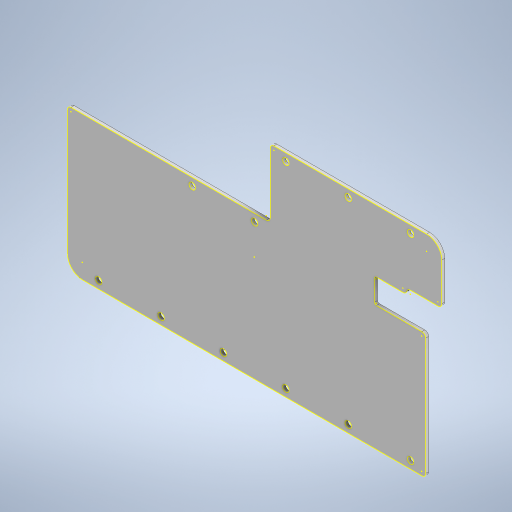
# Autodesk Inventor part: Class-D RevA Board Outline
Saved by Autodesk Inventor 2024 (Build 280153000, 153)
## iProperties
Created: 2023-08-05
Part Number: Class-D RevA Board Outline
Material: Generic
Document SubType Name: Modeling
Designer: Ishaan
Density: 1 g/cm^3
Appearance: Default
Author: Ishaan
Autodesk Inventor part; units mm, degrees
ref_plane "YZ Plane" through (0, 0, 0) normal (1, 0, 0) x (0, 1, 0)
ref_plane "XZ Plane" through (0, 0, 0) normal (0, 1, 0) x (-1, 0, 0)
ref_plane "XY Plane" through (0, 0, 0) normal (0, 0, 1) x (1, 0, 0)
sketch "Sketch1" plane through (0, 0, 0) normal (0, 0, 1) x (1, 0, 0)
  line L0 (-99, -56) -> (99, -56)
  line L1 (99, -56) -> (99, 56)
  line L2 (99, 56) -> (-99, 56)
  line L3 (-99, 56) -> (-99, -56)
  line L4 (-99, -56) -> (99, 56) construction
  line L5 (99, -56) -> (-99, 56) construction
  line L6 (-99, -56) -> (8.25, -56)
  line L7 (8.25, -56) -> (8.25, 20)
  line L8 (8.25, 20) -> (-99, 20)
  line L9 (-99, 20) -> (-99, -56)
  line L10 (8.25, 20) -> (8.25, 56)
  point P0 (0, 0)
  dimension "d0" = 112
  dimension "d1" = 198
  dimension "d3" = 76
  dimension "d50" = 8.25
  constraints: 22 end point, 4 parallel, 3 perpendicular, 2 horizontal, 2 midpoint, 1 point on line
  measures "d0" distance of L0.end L1.end
  measures "d1" distance of L1.end L2.end
  measures "d3" distance of L6.end L7.end
  measures "d50" distance from line of L10 point (0, 0)
extrude "Extrusion1" add sketch "Sketch1" along normal blind 1.6 contours L3 L8 L7 L0 | L7 L10 L2 L1 L0
sketch "Sketch2" plane through (0, 0, 1.6) normal (0, 0, 1) x (1, 0, 0)
  line L0 (-99, -56) -> (99, -56) projected
  line L1 (-99, 20) -> (-99, -56) projected
  line L2 (99, 56) -> (8.25, 56) projected
  line L3 (99, -56) -> (99, 56) projected
  line L4 (8.25, 20) -> (-99, 20) projected
  line L5 (-16.5, -52) -> (16.5, -52) construction
  line L6 (-49.5, -52) -> (-16.5, -52) construction
  point P0 (0, 0)
  point P1 (-82.5, -52)
  point P2 (49.5, -52)
  point P3 (-82.5, 52)
  point P4 (-49.5, 52)
  point P5 (-16.5, 52)
  point P6 (16.5, 52)
  point P7 (49.5, 52)
  point P8 (82.5, -52)
  point P9 (82.5, 52)
  point P10 (-33, 16)
  point P11 (0, 16)
  point P12 (0, -52)
  point P13 (-33, -52)
  point P14 (-99, 56)
  dimension "d6" = 4
  dimension "d9" = 33
  dimension "d12" = 104
  dimension "d15" = 4
  dimension "d17" = 16.5
  dimension "d18" = 16.5
  dimension "d26" = 4
  constraints: 4 end point, 3 horizontal, 2 midpoint, 2 vertical alignment, 1 coincident, 1 horizontal alignment, 1 vertical, 11 other
  measures "d6" distance from line of point (-82.5, -52) L0
  measures "d9" distance of point (-82.5, -52) L6.start
  measures "d12" distance of point (-82.5, -52) point (-82.5, 52)
  measures "d15" distance from line of L2 point (-82.5, 52)
  measures "d17" distance from line of point (-82.5, -52) L1
  measures "d18" distance from line of point (82.5, -52) L3
  measures "d26" distance from line of L4 point (-33, 16)
hole "Hole1" at (-82.5, -52, 1.6) at (-49.5, -52, 1.6) at (-16.5, -52, 1.6) at (16.5, -52, 1.6) at (49.5, -52, 1.6) at (-82.5, 52, 1.6) at (-49.5, 52, 1.6) at (-16.5, 52, 1.6) at (16.5, 52, 1.6) at (49.5, 52, 1.6) at (82.5, -52, 1.6) at (82.5, 52, 1.6) at (-33, 16, 1.6) at (0, 16, 1.6) direction (0, 0, -1) diameter 3.4 end through all
sketch "Sketch3" plane through (0, 0, 1.6) normal (0, 0, 1) x (1, 0, 0)
  circle A0 centre (0, 16) radius 1.7 projected
  circle A1 centre (-33, 16) radius 1.7 projected
  circle A2 centre (82.5, 52) radius 1.7 projected
  circle A3 centre (82.5, -52) radius 1.7 projected
  circle A4 centre (49.5, 52) radius 1.7 projected
  circle A5 centre (16.5, 52) radius 1.7 projected
  circle A6 centre (49.5, -52) radius 1.7 projected
  circle A7 centre (16.5, -52) radius 1.7 projected
  circle A8 centre (-16.5, -52) radius 1.7 projected
  circle A9 centre (-49.5, -52) radius 1.7 projected
  circle A10 centre (-82.5, -52) radius 1.7 projected
  line L0 (99, 56) -> (8.25, 56) projected
  line L1 (-99, 20) -> (-99, -56) projected
  line L2 (-99, -56) -> (99, -56) projected
  line L3 (99, -56) -> (99, 56) projected
  line L4 (99, 26) -> (0, 26) construction
  line L5 (99, 10) -> (-99, 10) construction
  line L6 (90.5, -56) -> (90.5, 10)
  line L7 (99, 26) -> (80.5, 26)
  line L8 (80.5, 26) -> (80.5, 10)
  line L9 (90.5, 10) -> (80.5, 10)
  line L10 (63.5, 10) -> (80.5, 10)
  line L11 (80.5, 10) -> (80.5, 23)
  line L12 (80.5, 23) -> (63.5, 23)
  line L13 (63.5, 23) -> (63.5, 10)
  line L14 (63.5, 10) -> (80.5, 23) construction
  line L15 (80.5, 10) -> (63.5, 23) construction
  line L16 (8.25, 56) -> (8.25, 20) projected
  line L17 (8.25, 20) -> (-99, 20) projected
  point P0 (0, 0)
  point P1 (82.5, 30)
  point P2 (72, 16.5)
  dimension "d27" = 30
  dimension "d29" = 4
  dimension "d30" = 8
  dimension "d31" = 4
  dimension "d32" = 4
  dimension "d33" = 2
  dimension "d36" = 72.5
  dimension "d37" = 17
  dimension "d38" = 13
  constraints: 24 end point, 8 point on line, 3 perpendicular, 2 midpoint, 2 parallel, 2 vertical, 1 collinear, 1 horizontal, 1 vertical alignment
  measures "d27" distance between parallel lines of L0 L4
  measures "d29" distance from line of L2 A3.centre
  measures "d30" distance from line of L6 A3.centre
  measures "d31" distance from line of L4 point (82.5, 30)
  measures "d32" distance from line of L0 A2.centre
  measures "d33" distance from line of L8 point (82.5, 30)
  measures "d36" distance from line of L2 point (72, 16.5)
  measures "d37" distance between parallel lines of L8 L13
  measures "d38" distance between parallel lines of L12 L10
extrude "Extrusion2" cut sketch "Sketch3" against normal through all contours L3 L2 L6 L9 L8 L7 | L8 L10 L13 L12
fillet "Fillet1" radius 8 2 edges at (-99, -56, 0.8) (99, 56, 0.8)
fillet "Fillet2" radius 2 8 edges at (90.5, 10, 0.8) (8.25, 20, 0.8) (80.5, 23, 0.8) (80.5, 26, 0.8) (99, 26, 0.8) (-99, 20, 0.8) (8.25, 56, 0.8) (90.5, -56, 0.8)
fillet "Fillet3" radius 1 2 edges at (63.5, 23, 0.8) (63.5, 10, 0.8)
sketch "Sketch5" plane through (0, 0, 1.6) normal (0, 0, 1) x (1, 0, 0)
  circle A0 centre (0, 16) radius 1.7 projected
  circle A1 centre (-33, 16) radius 1.7 projected
  circle A2 centre (82.5, 52) radius 1.7 projected
  circle A3 centre (82.5, -52) radius 1.7 projected
  circle A4 centre (49.5, 52) radius 1.7 projected
  circle A5 centre (16.5, 52) radius 1.7 projected
  circle A6 centre (49.5, -52) radius 1.7 projected
  circle A7 centre (16.5, -52) radius 1.7 projected
  circle A8 centre (-16.5, -52) radius 1.7 projected
  circle A9 centre (-49.5, -52) radius 1.7 projected
  circle A10 centre (-82.5, -52) radius 1.7 projected
  arc A11 (88.5, -56) -> (90.5, -54) centre (88.5, -54) ccw projected
  line L0 (90.5, -54) -> (90.5, 8) projected
  arc A12 (90.5, 8) -> (88.5, 10) centre (88.5, 8) ccw projected
  line L1 (88.5, 10) -> (64.5, 10) projected
  arc A13 (63.5, 11) -> (64.5, 10) centre (64.5, 11) ccw projected
  line L2 (63.5, 11) -> (63.5, 22) projected
  arc A14 (64.5, 23) -> (63.5, 22) centre (64.5, 22) ccw projected
  line L3 (64.5, 23) -> (78.5, 23) projected
  arc A15 (78.5, 23) -> (80.4365, 24.5) centre (78.5, 25) ccw projected
  arc A16 (82.373, 26) -> (80.4365, 24.5) centre (82.373, 24) ccw projected
  line L4 (82.373, 26) -> (97, 26) projected
  arc A17 (97, 26) -> (99, 28) centre (97, 28) ccw projected
  line L5 (99, 28) -> (99, 48) projected
  arc A18 (99, 48) -> (91, 56) centre (91, 48) ccw projected
  line L6 (91, 56) -> (10.25, 56) projected
  arc A19 (10.25, 56) -> (8.25, 54) centre (10.25, 54) ccw projected
  line L7 (8.25, 54) -> (8.25, 22) projected
  arc A20 (6.25, 20) -> (8.25, 22) centre (6.25, 22) ccw projected
  line L8 (6.25, 20) -> (-97, 20) projected
  arc A21 (-97, 20) -> (-99, 18) centre (-97, 18) ccw projected
  line L9 (-99, 18) -> (-99, -48) projected
  arc A22 (-99, -48) -> (-91, -56) centre (-91, -48) ccw projected
  line L10 (-91, -56) -> (88.5, -56) projected
  point P0 (0, 0)
equation "\"d15\" = d6"
equation "\"d18\" = d17"
equation "\"d31\" = d32"
body "Solid1"
